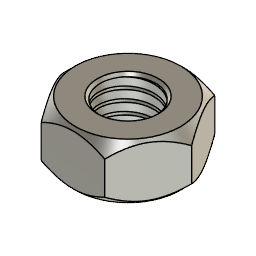
M6_hex_nut (Autodesk Fusion 360 design; units mm, degrees)
part number: 2026-04-25-09-47-30-495
Autodesk Fusion 360 part; units mm, degrees
sketch "Hex Nut Shape" plane through (0, 0, 0) normal (0, 0, 1) x (1, 0, 0)
  line L0 (-2.8868, 5) -> (-5.7735, 0)
  line L1 (-5.7735, 0) -> (-2.8868, -5)
  line L2 (-2.8868, -5) -> (2.8868, -5)
  line L3 (2.8868, -5) -> (5.7735, 0)
  line L4 (5.7735, 0) -> (2.8868, 5)
  line L5 (2.8868, 5) -> (-2.8868, 5)
  dimension "d3" = 10
  measures "d3" distance of L2 L5
extrude "Extrude1" add sketch "Hex Nut Shape" along normal blind 5
sketch "Chamfer Outline" plane through (0, 0, 0) normal (0, 1, 0) x (1, 0, 0)
  line L0 (2.8868, 0) -> (5.7735, 0)
  line L1 (5.7735, 0) -> (5.7735, -5)
  line L2 (5.7735, -5) -> (2.8868, -5)
  line L3 (2.8868, -5) -> (2.8868, 0)
  line L4 (-2.8868, 0) -> (2.8868, 0)
  line L5 (2.8868, 0) -> (2.8868, -5)
  line L6 (2.8868, -5) -> (-2.8868, -5)
  line L7 (-2.8868, -5) -> (-2.8868, 0)
  line L8 (-5.7735, 0) -> (-2.8868, 0)
  line L9 (-2.8868, 0) -> (-2.8868, -5)
  line L10 (-2.8868, -5) -> (-5.7735, -5)
  line L11 (-5.7735, -5) -> (-5.7735, 0)
  line L12 (5.7735, -5) -> (4.7735, -5)
  line L13 (5.7735, -5) -> (5.7735, -4)
  line L14 (5.7735, 0) -> (5.7735, -1)
  line L15 (5.7735, 0) -> (4.7735, 0)
  line L16 (4.7735, -5) -> (5.7735, -4)
  line L17 (5.7735, -1) -> (4.7735, 0)
  dimension "d11" = 1
  dimension "d12" = 1
  dimension "d13" = 1
  dimension "d14" = 1
  constraint coincident L1.end L2.start
  constraint perpendicular L1 L12
  constraint coincident L1 L13.end
  constraint coincident L0.end L1.start
  constraint perpendicular L2 L14
  constraint perpendicular L14 L15
  measures "d11" distance of L1.end L12.end
  measures "d12" distance of L1.end L13.end
  measures "d13" distance of L0.end L14.end
  measures "d14" distance of L0.end L15.end
revolve "Revolve1" cut sketch "Chamfer Outline" angle 360 about axis through (0, 0, 1.75) along (0, 0, 1) contours L0 L1 L14 L15 L17 | L1 L2 L12 L13 L16
hole "Hole1" at (0, 0, 5) direction (0, 0, -1) diameter 6 end through all
chamfer "Chamfer1" distance 0.25 angle 45 2 edges at (-2.797, 1.0848, 5) (-2.797, -1.0848, 0)
thread "Thread1" "ISO Metric profile 6.0 M6x1 M6x1 6H" major diameter 6.147 minor diameter 5.035 pitch 1 angle 60 modelled right hand crest width 0.2748 on face at (0.1495, -2.9963, 3.25) crest through (2.5175, 0, 4.5)
equation "width_across_flats = 10 mm" comment "An M6 hex nut has a width across the flats of 10 mm."
equation "thickness = 5 mm" comment "An M6 hex nut has a thickness of 5 mm."
equation "d3 = width_across_flats"
equation "d4 = thickness"
equation "chamfer_side_length = 1 mm" comment "Chamfer on the outside top and bottom of the hex nut."
equation "d11 = chamfer_side_length"
equation "d12 = chamfer_side_length"
equation "d13 = chamfer_side_length"
equation "d14 = chamfer_side_length"
equation "d16 = hole_diameter"
equation "hole_diameter = 6 mm" comment "An M6 hex nut has a hole diameter of 6 mm."
equation "hole_chamfer = 0.25 mm" comment "Chamfer on the inside of the hex nut thread hole."
equation "d20 = hole_chamfer"
named bodies: "M6 Hex Nut"
